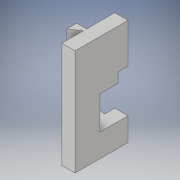
# Autodesk Inventor part: Inner Rails 2
Saved by Autodesk Inventor 2019 (Build 230136000, 136)
## iProperties
Created: 2019-03-02
Part Number: Inner Rails 2
Material: Generic
Document SubType Name: Modeling
Designer: Jared
Density: 1 g/cm^3
Appearance: Default
Author: Jared
Autodesk Inventor part; units mm, degrees
ref_plane "YZ Plane" through (0, 0, 0) normal (1, 0, 0) x (0, 1, 0)
ref_plane "XZ Plane" through (0, 0, 0) normal (0, 1, 0) x (-1, 0, 0)
ref_plane "XY Plane" through (0, 0, 0) normal (0, 0, 1) x (1, 0, 0)
sketch "Sketch1" plane through (0, 0, 0) normal (0, 1, 0) x (-1, 0, 0)
  line L0 (0, 0) -> (0, -16)
  line L1 (0, -16) -> (4, -16)
  line L2 (0, 0) -> (4, 0)
  line L3 (4, 0) -> (4, -6.5)
  line L4 (4, -16) -> (4, -13)
  line L5 (4, -13) -> (7, -13)
  line L6 (7, -13) -> (7, -4.5)
  line L7 (7, -4.5) -> (4, -6.5)
  dimension "d0" = 16
  dimension "d1" = 4
  dimension "d2" = 6.5
  dimension "d3" = 3
  dimension "d4" = 3
  dimension "d5" = 8.5
  constraints: 16 end point, 3 vertical, 2 parallel, 2 perpendicular, 1 horizontal
  measures "d0" distance of L0.start L0.end
  measures "d1" distance of L0.end L1.end
  measures "d2" distance of L2.end L3.end
  measures "d3" distance of L1.end L4.end
  measures "d4" distance of L4.end L5.end
  measures "d5" distance of L5.end L6.end
extrude "Extrusion1" add sketch "Sketch1" along normal blind 32
sketch "Sketch2" plane through (-7, 0, -13) normal (-1, 0, 0) x (0, 0, 1)
  line L0 (0, 0) -> (8.5, 0) projected
  line L1 (8.5, 0) -> (8.5, 32) projected
  line L2 (0, 32) -> (8.5, 32) projected
  line L3 (0, 0) -> (0, 32) projected
  line L4 (0, 32) -> (8.5, 32) projected
  line L5 (5.5, 32) -> (5.5, 7)
  line L6 (5.5, 7) -> (0, 7)
  line L7 (0, 0) -> (0, 32) projected
  point P0 (13, 0)
  dimension "d8" = 25
  dimension "d9" = 5.5
  constraints: 4 end point, 2 point on line, 1 perpendicular, 1 vertical
  measures "d8" distance of L5.start L5.end
  measures "d9" distance of L5.end L6.end
extrude "Extrusion2" cut sketch "Sketch2" against normal blind 3 contours L3 L2 L5 L6
sketch "Sketch3" plane through (-4, 0, -16) normal (-1, 0, 0) x (0, 0, 1)
  line L0 (0, 0) -> (3, 0) projected
  line L1 (3, 0) -> (3, 7) projected
  line L2 (8.5, 7) -> (3, 7) projected
  line L3 (8.5, 32) -> (8.5, 7) projected
  line L4 (0, 32) -> (8.5, 32) projected
  line L5 (0, 0) -> (0, 32) projected
  line L6 (0, 0) -> (0, 32) projected
  line L7 (0, 32) -> (0, 20)
  line L8 (0, 20) -> (3, 20)
  line L9 (8.5, 32) -> (8.5, 7) projected
  line L10 (0, 32) -> (8.5, 32) projected
  line L11 (3, 32) -> (3, 17)
  line L12 (3, 17) -> (8.5, 17)
  line L13 (0, 0) -> (0, 32) projected
  line L14 (0, 7) -> (3, 7)
  point P0 (16, 0)
  dimension "d12" = 12
  dimension "d13" = 15
  dimension "d14" = 3
  constraints: 10 end point, 5 point on line, 4 perpendicular
  measures "d12" distance of L4.start L7.end
  measures "d13" distance of L11.start L11.end
  measures "d14" distance between parallel lines of L5 L11
extrude "Extrusion3" cut sketch "Sketch3" against normal blind 4 contours L5 L8 L11 L12 L3 L2 L14
body "Solid1"
